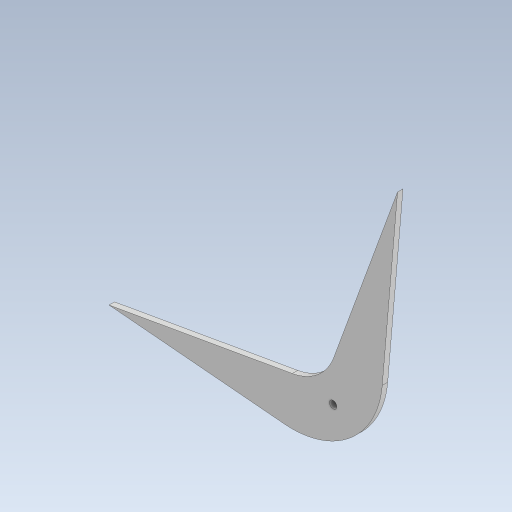
# Autodesk Inventor part: sus_1
Saved by Autodesk Inventor 2023 (Build 270158000, 158)
## iProperties
Created: 2023-06-07
Part Number: sus_1
Material: 一般
Document SubType Name: Modeling
Designer: JOU
Density: 1 g/cm^3
Appearance: 預設
Author: JOU
Autodesk Inventor part; units mm, degrees
ref_plane "YZ Plane" through (0, 0, 0) normal (1, 0, 0) x (0, 1, 0)
ref_plane "XZ Plane" through (0, 0, 0) normal (0, 1, 0) x (-1, 0, 0)
ref_plane "XY Plane" through (0, 0, 0) normal (0, 0, 1) x (1, 0, 0)
sketch "草圖1" plane through (0, 0, 0) normal (0, 0, 1) x (1, 0, 0)
  arc A0 (-17.0574, -3.0077) -> (5.924, 16.276) centre (-22.2668, 26.5366) ccw
  line L0 (5.924, 16.276) -> (41.0424, 112.7631)
  line L1 (-118.1769, -20.8378) -> (-17.0574, -3.0077)
  line L2 (-118.1769, -20.8378) -> (-21.5765, -29.2892)
  arc A1 (-21.5765, -29.2892) -> (32.591, 16.1627) centre (-17.2188, 20.5205) ccw
  line L3 (32.591, 16.1627) -> (41.0424, 112.7631)
  circle A2 centre (5.5072, -6.5632) radius 2
  point P0 (0, 0)
  dimension "d0" = 50
  dimension "d1" = 4
  dimension "d2" = 25
  dimension "d3" = 25
  constraints: 8 end point, 4 point on circle, 3 centre point, 2 perpendicular, 2 tangent, 8 other
  measures "d0" radius of A1
  measures "d1" diameter of A2
  measures "d2" distance from line of L3 A2.centre
  measures "d3" distance from line of L2 A2.centre
extrude "擠出1" add sketch "草圖1" along normal blind 3
equation "\"d3\" = d2"
